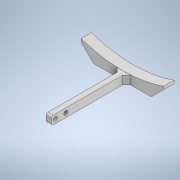
# Autodesk Inventor part: tete_statique
Saved by Autodesk Inventor 2020 (Build 240168000, 168)
## iProperties
Created: 2019-12-28
Part Number: tete_statique
Material: Générique
Document SubType Name: Modeling
Designer: bapti
Density: 1 g/cm^3
Appearance: Par défaut
Author: bapti
Autodesk Inventor part; units mm, degrees
ref_plane "YZ Plane" through (0, 0, 0) normal (1, 0, 0) x (0, 1, 0)
ref_plane "XZ Plane" through (0, 0, 0) normal (0, 1, 0) x (-1, 0, 0)
ref_plane "XY Plane" through (0, 0, 0) normal (0, 0, 1) x (1, 0, 0)
sketch "Esquisse1" plane through (0, 0, 0) normal (0, 0, 1) x (1, 0, 0)
  line L0 (0, 0) -> (0, 15)
  line L1 (0, 0) -> (80, 0)
  line L2 (80, 0) -> (80, 15)
  arc A0 (0, 15) -> (80, 15) centre (40, 129.2471) ccw
  line L3 (0, 8.2) -> (80, 8.2) construction
  line L4 (40, 0) -> (40, 8.2) construction
  dimension "d0" = 15
  dimension "d1" = 80
  dimension "d28" = 8.2
  constraints: 10 end point, 2 midpoint, 2 perpendicular, 2 point on circle, 2 point on line, 1 centre point, 1 horizontal, 1 parallel, 1 tangent, 1 vertical
  measures "d0" distance of L0.start L0.end
  measures "d1" distance of L0.start L1.end
  measures "d28" distance of L4.start L4.end
extrude "Extrusion1" add sketch "Esquisse1" along normal blind 10
sketch "Esquisse2" plane through (0, 0, 10) normal (0, 0, 1) x (1, 0, 0)
  line L0 (0, 0) -> (80, 0) projected
  line L1 (39, 0) -> (44, 0)
  line L2 (44, 0) -> (44, 8.2)
  line L3 (44, 8.2) -> (39, 8.2)
  line L4 (39, 8.2) -> (39, 0)
  line L5 (0, 15) -> (0, 0) projected
  line L6 (0, 8.2) -> (80, 8.2) construction
  line L7 (80, 0) -> (80, 15) projected
  arc A0 (0, 15) -> (80, 15) centre (40, 129.2471) ccw projected
  line L8 (40, 0) -> (40, 8.2) construction
  dimension "d6" = 5
  dimension "d9" = 80
  dimension "d56" = 4
  constraints: 12 end point, 3 point on line, 2 horizontal, 2 parallel, 1 collinear, 1 midpoint, 1 perpendicular, 1 point on circle, 1 tangent
  measures "d6" distance of L2.end L3.end
  measures "d9" distance of L0.start L0.end
  measures "d56" distance between parallel lines of L2 L8
extrude "Extrusion2" add sketch "Esquisse2" along normal blind 72.9 contours L4 L3 L2 L0
sketch "Esquisse8" plane through (39, 0, 10) normal (-1, 0, 0) x (0, 0, 1)
  circle A0 centre (69.075, 4.1) radius 2
  circle A1 centre (58.975, 4.1) radius 2
  line L0 (0, 8.2) -> (72.9, 8.2) projected
  line L1 (0, 0) -> (72.9, 0) projected
  line L2 (72.9, 8.2) -> (72.9, 0) projected
  point P0 (-10, 0)
  dimension "d45" = 10.1
  dimension "d46" = 4
  dimension "d47" = 4
  dimension "d48" = 8.2
  dimension "d49" = 4.1
  dimension "d50" = 4.1
  dimension "d51" = 3.825
  constraints: 2 centre point
  measures "d45" distance of A0.centre A1.centre
  measures "d46" diameter of A0
  measures "d47" diameter of A1
  measures "d48" distance between parallel lines of L0 L1
  measures "d49" distance from line of L1 A1.centre
  measures "d50" distance from line of L1 A0.centre
  measures "d51" distance from line of L2 A0.centre
extrude "Extrusion8" cut sketch "Esquisse8" against normal up to surface (5 mm away)
chamfer "Chanfrein1" distance 4 angle 45 2 edges at (39, 4.1, 10) (44, 4.1, 10)
chamfer "Chanfrein2" distance 12 angle 45 2 edges at (0, 0, 5) (80, 0, 5)
fillet "Congé1" radius 2 2 edges at (41.5, 8.2, 82.9) (41.5, 0, 82.9)
equation "\"d47\" = d46"
equation "\"d49\" = 0.5 * d48"
equation "\"d50\" = d49"
